Autodesk Fusion 360 part; units mm, degrees
(part 2 of 2)
sketch "Sketch1 (2)" plane through (0, 0, -285) normal (0, 0, -1) x (-1, 0, 0) in component "stage"
  line L0 (-20, 20) -> (20, 20)
  line L1 (20, 20) -> (20, -20)
  line L2 (20, -20) -> (-20, -20)
  line L3 (-20, -20) -> (-20, 20)
  line L4 (-20, 20) -> (20, -20) construction
  line L5 (20, 20) -> (-20, -20) construction
  dimension "d98" = 40
  constraint horizontal L0
  constraint perpendicular L0 L1
  constraint parallel L0 L2
  constraint parallel L1 L3
  constraint coincident L4 origin
  constraint coincident L5 origin
  constraint equal L1 L2
  measures "d98" distance of L0.end L1.end
extrude "Extrude1" [suppressed] in component "stage"
ref_plane "WorkPlane2" through (0, 0, -305) normal (0, 0, -1) x (-1, 0, 0) in component "rotate"
sketch "Sketch1 (3)" plane through (0, 0, 0) normal (0, 0, 1) x (0, 1, 0) in component "decoupler"
  line L0 (-20, 40) -> (-20, 0) construction
  line L1 (-20, 0) -> (20, 0) construction
  line L2 (20, 40) -> (-20, 40) construction
  line L3 (114.24, 2.9982) -> (46.1305, 2.9982) construction
  line L4 (46.1305, -6.808) -> (114.24, -16.8596) construction
  line L5 (46.1305, 9.2293) -> (114.24, 22.856) construction
  line L6 (46.1305, 9.2293) -> (0, 0) construction
  line L7 (46.1305, 2.9982) -> (0, 0) construction
  line L8 (46.1305, -6.808) -> (0, 0) construction
  line L9 (46.1305, -15.3931) -> (0, 0) construction
  line L10 (46.1305, -15.3931) -> (114.24, -38.1203)
  line L11 (46.1305, 17.8145) -> (0, 0) construction
  line L12 (46.1305, 17.8145) -> (114.24, 44.1167)
  line L13 (119.5552, -38.1203) -> (114.24, -38.1203)
  line L14 (114.24, -38.1203) -> (114.24, 44.1167)
  line L15 (114.24, 44.1167) -> (119.5552, 44.1167)
  line L16 (119.5552, 44.1167) -> (119.5552, -38.1203)
  line L17 (114.24, -37.0661) -> (46.1305, -14.3389)
  line L18 (46.1305, -15.3931) -> (46.1305, -14.3389)
  line L19 (114.24, 43.0447) -> (46.1305, 16.7425)
  line L20 (46.1305, 8.7194) -> (114.24, 22.3461) construction
  line L21 (114.24, 23.3659) -> (46.1305, 9.7392) construction
  line L22 (46.1305, 3.4982) -> (114.24, 3.4982)
  line L23 (114.24, 2.4982) -> (46.1305, 2.4982)
  line L24 (46.1305, -6.3026) -> (114.24, -16.3542) construction
  line L25 (46.1305, -7.3134) -> (114.24, -17.365) construction
  line L26 (80.1853, -11.3284) -> (80.1853, -12.3392) construction
  line L27 (80.1853, 3.4982) -> (80.1853, 2.4982) construction
  line L28 (80.1853, 16.5526) -> (80.1853, 15.5327) construction
  line L29 (46.1305, 17.8145) -> (46.1305, 16.7425)
  line L30 (46.1305, 9.7392) -> (46.1305, 8.7194)
  line L31 (46.1305, 3.4982) -> (46.1305, 2.4982)
  line L32 (46.1305, -6.3026) -> (46.1305, -7.3134)
  line L33 (46.1305, -14.3389) -> (46.1305, -15.3931)
  line L34 (46.1305, 0) -> (46.1305, 40)
  line L35 (46.1305, 0) -> (20, 0)
  line L36 (20, 0) -> (20, 40)
  line L37 (20, 40) -> (46.1305, 40)
  line L38 (46.1305, 40) -> (46.1305, 0)
  arc A0 (80.1284, 29.8716) -> (79.7736, 30.8066) centre (0, 0) ccw construction
  arc A1 (83.9502, 16.286) -> (83.8536, 16.7766) centre (0, 0) ccw construction
  point P0 (80.1853, -11.8338)
  point P1 (80.1853, 2.9982)
  point P2 (80.1853, 16.0426)
  dimension "roatate_flex_thick" = 1
  dimension "d102" = 1
  dimension "d109" = 1
  dimension "d111" = 1
  dimension "d112" = 1
  constraint parallel L5 L6
  constraint parallel L4 L8
  constraint coincident L6.end L7.end
  constraint parallel L9 L10
  constraint parallel L11 L12
  constraint symmetric L3 L10.end L12.end
  constraint symmetric L3 L4.end L5.end
  constraint horizontal L13
  constraint vertical L14
  constraint horizontal L15
  constraint vertical L16
  constraint coincident L10.end L13.end
  constraint coincident L5.end L14
  constraint coincident L3.start L14
  constraint coincident L4.end L14
  constraint coincident L14 L17.start
  constraint parallel L10 L17
  constraint coincident L14 L19.start
  constraint parallel L12 L19
  constraint midpoint L4 P0
  constraint midpoint L3 P1
  constraint midpoint L5 P2
  constraint coincident L14 L20.end
  constraint parallel L5 L20
  constraint coincident L14 L21.start
  constraint parallel L5 L21
  constraint coincident L14 L22.end
  constraint coincident L14 L23.start
  constraint coincident L14 L24.end
  constraint parallel L4 L24
  constraint coincident L14 L25.end
  constraint parallel L4 L25
  constraint midpoint L24 L26.start
  constraint coincident L25 L26.end
  constraint midpoint L25 L26.end
  constraint midpoint P0 L26
  constraint parallel L3 L22
  constraint midpoint L22 L27.start
  constraint midpoint L23 L27.end
  constraint midpoint L21 L28.start
  constraint midpoint L20 L28.end
  constraint coincident P1 L27
  constraint midpoint P1 L27
  constraint midpoint P2 L28
  constraint coincident L12.end L14.end
  constraint vertical L34
  constraint coincident L9.start L34
  constraint coincident L25.start L34
  constraint coincident L23.end L34
  constraint coincident L22.start L34
  constraint coincident L20.start L34
  constraint coincident L21.end L34
  constraint coincident L11.start L34
  constraint coincident L19.end L34
  constraint coincident L24.start L34
  constraint coincident L17.end L34
  constraint horizontal L35
  constraint vertical L36
  constraint horizontal L37
  constraint vertical L38
  constraint coincident L2.start L36.end
  constraint coincident L34.end L37
  constraint coincident L1.end L35
  constraint coincident L12 A0.end
  constraint coincident L19 A0.start
  constraint coincident L5 A1.end
  constraint coincident L20 A1.start
  measures "roatate_flex_thick" distance of L10 L17
  measures "d102" distance of L12 L19
  measures "d109" distance of L20 L21
  measures "d111" distance of L22 L23
  measures "d112" distance of L24 L25
extrude "Extrude1'" [suppressed] in component "decoupler"
fillet "Fillet1" [suppressed] in component "decoupler"
component "xy" placed x (1, 0, 0) y (0, 1, 0) z (0, 0, 1) at (0, 0, 0)
component "rotate" placed x (1, 0, 0) y (0, 1, 0) z (0, 0, 1) at (0, 0, 0)
component "frame" placed x (1, 0, 0) y (0, 1, 0) z (0, 0, 1) at (0, 0, 0)
component "top(z)" placed x (1, 0, 0) y (0, 1, 0) z (0, 0, 1) at (0, 0, 0)
component "scrue" placed x (1, 0, 0) y (0, 1, 0) z (0, 0, 1) at (0, 0, 0)
component "main xy flex" placed x (1, 0, 0) y (0, 1, 0) z (0, 0, 1) at (0, 0, 0) in component "xy"
equation "travle_xy = 15 mm"
equation "ofset_xy_travle = 2 mm"
equation "stage_size = 40 mm"
equation "zy_suqare_box = 220 mm"
equation "zy_flex_thicknes = -1.8 mm"
equation "xy_flex_down_extrude = 50 mm"
equation "stage_xy_intermideaat_body = 10 mm"
equation "d47 = stage_size"
equation "d48 = ofset_xy_travle + travle_xy"
equation "d56 = d64 / 10"
equation "d57 = zy_suqare_box / 2"
equation "d59 = -zy_flex_thicknes"
equation "d60 = zy_flex_thicknes"
equation "d61 = -zy_flex_thicknes"
equation "d62 = -zy_flex_thicknes"
equation "d64 = stage_size"
equation "d69 = -zy_flex_thicknes"
equation "d70 = d76"
equation "zy_flex_filet = 15 mm"
equation "d76 = ( 10 * 2.5 ) * 2.7 * 1 mm"
equation "d86 = stage_xy_intermideaat_body"
equation "d88 = stage_size"
equation "d92 = sqrt(( stage_size ) ^ 2 + ( stage_size ) ^ 2)"
equation "scrue_langth = 200 mm"
equation "d96 = scrue_top_stage"
equation "d98 = stage_size"
equation "d99 = stage_size"
equation "d102 = roatate_flex_thick"
equation "d109 = roatate_flex_thick"
equation "d111 = roatate_flex_thick"
equation "d112 = roatate_flex_thick"
equation "d113 = stage_size"
equation "decoupling_filit_radies = 3.0026285896 mm"
equation "d117 = d56"
